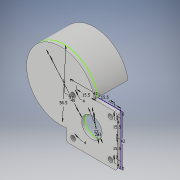
# Autodesk Inventor part: gear_retainer
Saved by Autodesk Inventor 2018 (Build 220112000, 112)
## iProperties
Created: 2018-04-23
Part Number: gear_retainer
Material: Generic
Document SubType Name: Modeling
Designer: guita
Density: 1 g/cm^3
Appearance: Default
Author: guita
Autodesk Inventor part; units mm, degrees
ref_plane "YZ Plane" through (0, 0, 0) normal (1, 0, 0) x (0, 1, 0)
ref_plane "XZ Plane" through (0, 0, 0) normal (0, 1, 0) x (-1, 0, 0)
ref_plane "XY Plane" through (0, 0, 0) normal (0, 0, 1) x (1, 0, 0)
sketch "Sketch1" plane through (0, 0, 0) normal (0, 0, 1) x (1, 0, 0)
  line L0 (0, 0) -> (42, 0)
  line L1 (42, 0) -> (42, 42)
  line L2 (42, 42) -> (0, 42)
  line L3 (0, 42) -> (0, 0)
  circle A0 centre (21, 21) radius 11.5
  line L4 (21, 42) -> (36.5, 42)
  line L5 (42, 21) -> (42, 36.5)
  line L6 (42, 21) -> (42, 5.5)
  line L7 (21, 42) -> (5.5, 42)
  circle A1 centre (5.5, 36.5) radius 2
  circle A2 centre (36.5, 36.5) radius 2
  circle A3 centre (36.5, 5.5) radius 2
  circle A4 centre (5.5, 5.5) radius 2
  line L8 (5.5, 38.5) -> (5.5, 34.5)
  line L9 (5.5, 7.5) -> (5.5, 5.5)
  circle A5 centre (21, 21) radius 12
  circle A6 centre (-5, 38) radius 18.5
  circle A7 centre (-5, 38) radius 22.5
  circle A8 centre (21, 21) radius 8.5
  arc A9 (22.9654, 42) -> (0, 10.196) centre (-5, 38) ccw
  arc A10 (17.9033, 42) -> (0, 15.294) centre (-5, 38) ccw
  circle A11 centre (-5, 38) radius 3
  dimension "d10" = 4
  dimension "d0" = 42
  dimension "d1" = 42
  dimension "d2" = 23
  dimension "d3" = 15.5
  dimension "d4" = 15.5
  dimension "d5" = 15.5
  dimension "d6" = 15.5
  dimension "d7" = 4
  dimension "d8" = 4
  dimension "d9" = 4
  dimension "d11" = 24
  dimension "d15" = 37
  dimension "d16" = 45
  dimension "d17" = 17
  dimension "d18" = 56.5
  dimension "d20" = 6
  constraints: 20 end point, 11 centre point, 8 point on line, 6 coincident, 6 point on circle, 3 midpoint, 2 parallel, 1 horizontal, 1 perpendicular, 1 vertical alignment, 2 other
  measures "d0" distance of L2.end L1.end
  measures "d1" distance of L1.end L0.end
  measures "d2" diameter of A0
  measures "d3" distance of L4.start L4.end
  measures "d4" distance of L5.start L5.end
  measures "d5" distance of L5.start L6.end
  measures "d6" distance of L4.start L7.end
  measures "d7" diameter of A1
  measures "d8" diameter of A2
  measures "d9" diameter of A3
  measures "d11" diameter of A5
  measures "d15" diameter of A6
  measures "d16" diameter of A7
  measures "d17" diameter of A8
  measures "d18" diameter of A9
  measures "d20" diameter of A11
extrude "Extrusion1" add sketch "Sketch1" along normal blind 3 contours L3 A7 A5 L2 L1 L0 | A9 L2 A10 L3 | A10 L2 A7 L3 | A7 L2 A6 L3 | L3 A6 L2 A7 A5 | A6 L2 L3 | L3 L2 A6 | A7 A0 A5 | A5 A7 A0 | A7 A0 | A0 A7 | A11
extrude "Extrusion2" add sketch "Sketch1" against normal blind 25 contours A9 L2 A10 L3
extrude "Extrusion3" add sketch "Sketch1" against normal blind 22 contours A11
fillet "Fillet1" radius 2 3 edges at (0, 0, 1.5) (42, 0, 1.5) (42, 42, 1.5)
body "Solid1"
